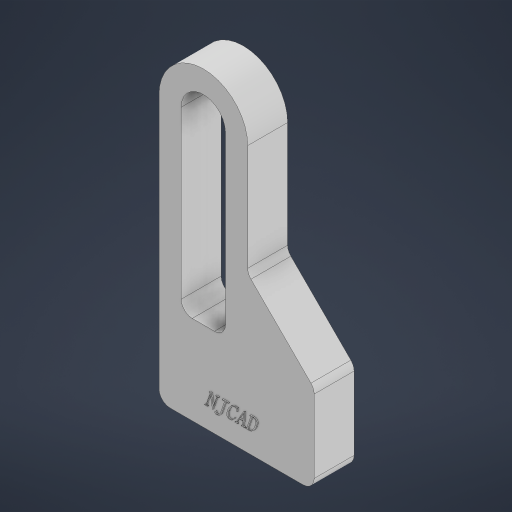
# Autodesk Inventor part: LOCK GUIDE
Saved by Autodesk Inventor 2023 (Build 270158000, 158)
## iProperties
Created: 2024-01-19
Part Number: LOCK GUIDE
Material: Generic
Document SubType Name: Modeling
Designer: User
Density: 1 g/cm^3
Appearance: Default
Author: User
Autodesk Inventor part; units mm, degrees
ref_plane "YZ Plane" through (0, 0, 0) normal (1, 0, 0) x (0, 1, 0)
ref_plane "XZ Plane" through (0, 0, 0) normal (0, 1, 0) x (-1, 0, 0)
ref_plane "XY Plane" through (0, 0, 0) normal (0, 0, 1) x (1, 0, 0)
sketch "Sketch1" plane through (0, 0, 0) normal (0, 0, 1) x (1, 0, 0)
  line L0 (0, 0) -> (70, 0)
  line L1 (70, 0) -> (70, 40)
  line L2 (0, 120) -> (0, 0)
  line L3 (70, 40) -> (40, 70)
  line L4 (40, 120) -> (40, 70)
  line L5 (10, 40) -> (30, 40)
  line L6 (30, 40) -> (30, 120)
  line L7 (10, 120) -> (10, 40)
  arc A0 (40, 120) -> (0, 120) centre (20, 120) ccw
  arc A1 (30, 120) -> (10, 120) centre (20, 120) ccw
  point P0 (20, 40)
  dimension "d8" = 120
  dimension "d13" = 30
  dimension "d15" = 30
  dimension "d16" = 40
  dimension "d17" = 20
  dimension "d20" = 40
  dimension "d21" = 70
  dimension "d22" = 80
  dimension "d23" = 20
  constraints: 16 end point, 4 point on circle, 3 perpendicular, 2 centre point, 2 horizontal, 2 parallel, 1 concentric, 1 horizontal alignment, 1 midpoint
  measures "d8" distance of L2.start L0.start
  measures "d13" distance from line of L3.end L1
  measures "d15" horizontal distance of L1.end L3.end
  measures "d16" distance between parallel lines of L6 L1
  measures "d17" distance of L5.start L5.end
  measures "d20" distance from line of point (20, 40) L0
  measures "d21" distance of L0.start L0.end
  measures "d22" distance of L7.start L5.start
  measures "d23" radius of A0
extrude "Extrusion1" add sketch "Sketch1" along normal blind 18
fillet "Fillet1" radius 5 6 edges at (40, 70, 9) (70, 40, 9) (10, 40, 9) (30, 40, 9) (0, 0, 9) (70, 0, 9)
sketch "Sketch2" plane through (0, 0, 18) normal (0, 0, 1) x (1, 0, 0)
  line L0 (20.8567, 15.7915) -> (48.2532, 15.7915) construction
  line L1 (48.2532, 15.7915) -> (48.2532, 8.4073) construction
  line L2 (48.2532, 8.4073) -> (20.8567, 8.4073) construction
  line L3 (20.8567, 8.4073) -> (20.8567, 15.7915) construction
  line L4 (24.9947, 10.9757) -> (25.066, 10.9757)
  line L5 (25.066, 10.9757) -> (26.484, 15.1494)
  spline S0 degree 2 poles (26.484, 15.1494) (26.5331, 15.2921) (26.435, 15.4348) (26.2566, 15.4348) knots 0 0 0 1 2 2 2
  line L6 (26.2566, 15.4348) -> (25.9712, 15.4348)
  line L7 (25.9712, 15.4348) -> (26.047, 15.6488)
  line L8 (26.047, 15.6488) -> (27.4739, 15.6488)
  line L9 (27.4739, 15.6488) -> (27.3981, 15.4348)
  line L10 (27.3981, 15.4348) -> (27.1127, 15.4348)
  spline S1 degree 2 poles (27.1127, 15.4348) (26.97, 15.4348) (26.7471, 15.2921) (26.698, 15.1494) knots 0 0 0 1 2 2 2
  line L11 (26.698, 15.1494) -> (24.794, 9.5488)
  line L12 (24.794, 9.5488) -> (24.58, 9.5488)
  line L13 (24.58, 9.5488) -> (23.6748, 14.864)
  line L14 (23.6748, 14.864) -> (23.6035, 14.864)
  line L15 (23.6035, 14.864) -> (21.967, 10.0482)
  spline S2 degree 2 poles (21.967, 10.0482) (21.9179, 9.9055) (22.0472, 9.7628) (22.1899, 9.7628) knots 0 0 0 1 2 2 2
  line L16 (22.1899, 9.7628) -> (22.4753, 9.7628)
  line L17 (22.4753, 9.7628) -> (22.404, 9.5488)
  line L18 (22.404, 9.5488) -> (20.9771, 9.5488)
  line L19 (20.9771, 9.5488) -> (21.0484, 9.7628)
  line L20 (21.0484, 9.7628) -> (21.3338, 9.7628)
  spline S3 degree 2 poles (21.3338, 9.7628) (21.5122, 9.7628) (21.7039, 9.9055) (21.7529, 10.0482) knots 0 0 0 1 2 2 2
  line L21 (21.7529, 10.0482) -> (23.4875, 15.1494)
  spline S4 degree 2 poles (23.4875, 15.1494) (23.5366, 15.2921) (23.4385, 15.4348) (23.2601, 15.4348) knots 0 0 0 1 2 2 2
  line L22 (23.2601, 15.4348) -> (23.0461, 15.4348)
  line L23 (23.0461, 15.4348) -> (23.1219, 15.6488)
  line L24 (23.1219, 15.6488) -> (24.1564, 15.6488)
  line L25 (24.1564, 15.6488) -> (24.9947, 10.9757)
  spline S5 degree 2 poles (29.9799, 15.1494) (30.029, 15.2921) (29.9309, 15.4348) (29.7525, 15.4348) knots 0 0 0 1 2 2 2
  line L26 (29.7525, 15.4348) -> (28.8964, 15.4348)
  line L27 (28.8964, 15.4348) -> (28.9722, 15.6488)
  line L28 (28.9722, 15.6488) -> (31.8973, 15.6488)
  line L29 (31.8973, 15.6488) -> (31.8215, 15.4348)
  line L30 (31.8215, 15.4348) -> (30.9654, 15.4348)
  spline S6 degree 2 poles (30.9654, 15.4348) (30.8227, 15.4348) (30.5997, 15.2921) (30.5507, 15.1494) knots 0 0 0 1 2 2 2
  line L31 (30.5507, 15.1494) -> (28.8295, 10.0839)
  spline S7 degree 2 poles (28.8295, 10.0839) (28.5619, 9.2991) (27.2599, 8.4073) (26.5108, 8.4073) knots 0 0 0 1 2 2 2
  spline S8 degree 2 poles (26.5108, 8.4073) (25.9757, 8.4073) (25.5521, 8.8353) (25.6457, 9.1207) knots 0 0 0 1 2 2 2
  spline S9 degree 2 poles (25.6457, 9.1207) (25.7215, 9.3348) (26.0426, 9.5488) (26.1853, 9.5488) knots 0 0 0 1 2 2 2
  spline S10 degree 2 poles (26.1853, 9.5488) (26.3636, 9.5488) (26.4929, 9.2991) (26.4305, 9.1207) knots 0 0 0 1 2 2 2
  spline S11 degree 2 poles (26.4305, 9.1207) (26.4082, 9.0494) (26.3369, 8.9424) (26.2388, 8.871) knots 0 0 0 1 2 2 2
  spline S12 degree 2 poles (26.2388, 8.871) (26.2744, 8.764) (26.5241, 8.657) (26.7382, 8.657) knots 0 0 0 1 2 2 2
  spline S13 degree 2 poles (26.7382, 8.657) (27.2019, 8.657) (27.9778, 9.2634) (28.2587, 10.0839) knots 0 0 0 1 2 2 2
  line L32 (28.2587, 10.0839) -> (29.9799, 15.1494)
  spline S14 degree 2 poles (32.4725, 9.4774) (31.4737, 9.4774) (30.8093, 10.9757) (31.3533, 12.581) knots 0 0 0 1 2 2 2
  spline S15 degree 2 poles (31.3533, 12.581) (31.8126, 13.9365) (33.6676, 15.7201) (34.7377, 15.7201) knots 0 0 0 1 2 2 2
  spline S16 degree 2 poles (34.7377, 15.7201) (34.9874, 15.7201) (35.2149, 15.6488) knots 0 0 0 1 1 1
  spline S17 degree 2 poles (35.2149, 15.6488) (35.4289, 15.5418) (35.6073, 15.5418) knots 0 0 0 1 1 1
  spline S18 degree 2 poles (35.6073, 15.5418) (35.7499, 15.5418) (35.9506, 15.6131) (36.0576, 15.7201) knots 0 0 0 1 2 2 2
  line L33 (36.0576, 15.7201) -> (35.848, 14.1505)
  line L34 (35.848, 14.1505) -> (35.6073, 14.0792)
  spline S19 degree 2 poles (35.6073, 14.0792) (35.6251, 14.757) (35.1524, 15.4704) (34.5817, 15.4704) knots 0 0 0 1 2 2 2
  spline S20 degree 2 poles (34.5817, 15.4704) (33.8325, 15.4704) (32.4547, 13.8295) (32.0445, 12.6166) knots 0 0 0 1 2 2 2
  spline S21 degree 2 poles (32.0445, 12.6166) (31.5941, 11.2967) (31.7992, 9.7985) (32.6197, 9.7985) knots 0 0 0 1 2 2 2
  spline S22 degree 2 poles (32.6197, 9.7985) (33.1904, 9.7985) (34.2874, 10.619) (34.6619, 11.2967) knots 0 0 0 1 2 2 2
  line L35 (34.6619, 11.2967) -> (34.8403, 11.1897)
  spline S23 degree 2 poles (34.8403, 11.1897) (34.4078, 10.4406) (33.1146, 9.4774) (32.4725, 9.4774) knots 0 0 0 1 2 2 2
  line L36 (38.2693, 11.8318) -> (36.6641, 11.8318)
  line L37 (36.6641, 11.8318) -> (35.8837, 10.4763)
  spline S24 degree 2 poles (35.8837, 10.4763) (35.7856, 10.2979) (35.7499, 10.1909) knots 0 0 0 1 1 1
  spline S25 degree 2 poles (35.7499, 10.1909) (35.7009, 10.0482) (35.7098, 9.7628) (35.9595, 9.7628) knots 0 0 0 1 2 2 2
  line L38 (35.9595, 9.7628) -> (36.0665, 9.7628)
  line L39 (36.0665, 9.7628) -> (35.9952, 9.5488)
  line L40 (35.9952, 9.5488) -> (34.6753, 9.5488)
  line L41 (34.6753, 9.5488) -> (34.7467, 9.7628)
  line L42 (34.7467, 9.7628) -> (34.8537, 9.7628)
  spline S26 degree 2 poles (34.8537, 9.7628) (34.9964, 9.7628) (35.2728, 9.9412) (35.3798, 10.1552) knots 0 0 0 1 2 2 2
  line L43 (35.3798, 10.1552) -> (38.626, 15.6131)
  line L44 (38.626, 15.6131) -> (39.2236, 15.7915)
  line L45 (39.2236, 15.7915) -> (38.6617, 10.1552)
  spline S27 degree 2 poles (38.6617, 10.1552) (38.6617, 9.9412) (38.8133, 9.7628) (38.956, 9.7628) knots 0 0 0 1 2 2 2
  line L46 (38.956, 9.7628) -> (39.063, 9.7628)
  line L47 (39.063, 9.7628) -> (38.9917, 9.5488)
  line L48 (38.9917, 9.5488) -> (37.4578, 9.5488)
  line L49 (37.4578, 9.5488) -> (37.5291, 9.7628)
  line L50 (37.5291, 9.7628) -> (37.6718, 9.7628)
  spline S28 degree 2 poles (37.6718, 9.7628) (37.8858, 9.7628) (38.0196, 9.9412) (38.0419, 10.0125) knots 0 0 0 1 2 2 2
  spline S29 degree 2 poles (38.0419, 10.0125) (38.091, 10.1552) (38.091, 10.2622) knots 0 0 0 1 1 1
  line L51 (38.091, 10.2622) -> (38.2693, 11.8318)
  line L52 (38.5993, 15.0067) -> (38.5636, 15.0067)
  line L53 (38.5636, 15.0067) -> (36.8067, 12.0459)
  line L54 (36.8067, 12.0459) -> (38.305, 12.0459)
  line L55 (38.305, 12.0459) -> (38.5993, 15.0067)
  spline S30 degree 2 poles (41.8232, 15.1494) (41.8722, 15.2921) (41.7741, 15.4348) (41.5958, 15.4348) knots 0 0 0 1 2 2 2
  line L56 (41.5958, 15.4348) -> (41.3817, 15.4348)
  line L57 (41.3817, 15.4348) -> (41.4575, 15.6488)
  line L58 (41.4575, 15.6488) -> (43.0628, 15.6488)
  spline S31 degree 2 poles (43.0628, 15.6488) (44.1687, 15.6488) (45.0025, 14.2219) (44.4942, 12.7236) knots 0 0 0 1 2 2 2
  spline S32 degree 2 poles (44.4942, 12.7236) (43.9368, 11.0827) (42.1309, 9.5488) (40.8823, 9.5488) knots 0 0 0 1 2 2 2
  line L59 (40.8823, 9.5488) -> (39.3484, 9.5488)
  line L60 (39.3484, 9.5488) -> (39.4198, 9.7628)
  line L61 (39.4198, 9.7628) -> (39.6695, 9.7628)
  spline S33 degree 2 poles (39.6695, 9.7628) (39.8478, 9.7628) (40.0396, 9.9055) (40.0886, 10.0482) knots 0 0 0 1 2 2 2
  line L62 (40.0886, 10.0482) -> (41.8232, 15.1494)
  spline S34 degree 2 poles (43.7896, 12.6523) (44.3114, 14.1862) (43.8075, 15.4348) (42.987, 15.4348) knots 0 0 0 1 2 2 2
  spline S35 degree 2 poles (42.987, 15.4348) (42.7373, 15.4348) (42.443, 15.2921) (42.394, 15.1494) knots 0 0 0 1 2 2 2
  line L63 (42.394, 15.1494) -> (40.6594, 10.0482)
  spline S36 degree 2 poles (40.6594, 10.0482) (40.6103, 9.9055) (40.7753, 9.7628) (40.9537, 9.7628) knots 0 0 0 1 2 2 2
  spline S37 degree 2 poles (40.9537, 9.7628) (41.7385, 9.7628) (43.21, 10.94) (43.7896, 12.6523) knots 0 0 0 1 2 2 2
  point P0 (0, 0)
  constraints: 2 other
emboss "Emboss1" sketch "Sketch2" operation add depth 0.5 direction (0, 0, -1)
body "Solid1"
